Autodesk Inventor part; units mm, degrees
(part 2 of 2)
sketch "Sketch14" plane through (0, 0, 0) normal (-1, 0, 0) x (0, 0, 1)
  line L0 (-9.7925, -188.2108) -> (9.4242, -188.2108) construction
  line L1 (9.4242, -188.2108) -> (9.4242, -196.9935) construction
  line L2 (9.4242, -196.9935) -> (-9.7925, -196.9935) construction
  line L3 (-9.7925, -196.9935) -> (-9.7925, -188.2108) construction
  line L4 (-9.4479, -191.3131) -> (-8.4204, -188.2651)
  line L5 (-8.4204, -188.2651) -> (-7.9214, -188.2651)
  line L6 (-7.9214, -188.2651) -> (-6.8939, -191.3131)
  line L7 (-6.8939, -191.3131) -> (-7.3212, -191.3131)
  line L8 (-7.3212, -191.3131) -> (-7.5979, -190.461)
  line L9 (-7.5979, -190.461) -> (-8.7612, -190.461)
  line L10 (-8.7612, -190.461) -> (-9.0379, -191.3131)
  line L11 (-9.0379, -191.3131) -> (-9.4479, -191.3131)
  line L12 (-7.709, -190.1152) -> (-8.1808, -188.6801)
  line L13 (-8.1808, -188.6801) -> (-8.6501, -190.1152)
  line L14 (-8.6501, -190.1152) -> (-7.709, -190.1152)
  line L15 (-4.2461, -191.3131) -> (-4.7722, -191.3131)
  line L16 (-4.7722, -191.3131) -> (-5.7355, -190.1003)
  line L17 (-5.7355, -190.1003) -> (-6.1998, -190.1003)
  line L18 (-6.1998, -190.1003) -> (-6.1998, -191.3131)
  line L19 (-6.1998, -191.3131) -> (-6.6049, -191.3131)
  line L20 (-6.6049, -191.3131) -> (-6.6049, -188.2651)
  line L21 (-6.6049, -188.2651) -> (-5.8195, -188.2651)
  spline S0 degree 2 poles (-5.8195, -188.2651) (-5.5576, -188.2651) (-5.2044, -188.3219) (-5.0439, -188.4257) knots 0 0 0 1 2 2 2
  spline S1 degree 2 poles (-5.0439, -188.4257) (-4.8833, -188.5294) (-4.6981, -188.853) (-4.6981, -189.0926) knots 0 0 0 1 2 2 2
  spline S2 degree 2 poles (-4.6981, -189.0926) (-4.6981, -189.426) (-5.0389, -189.878) (-5.3304, -189.9867) knots 0 0 0 1 2 2 2
  line L22 (-5.3304, -189.9867) -> (-4.2461, -191.3131)
  spline S3 degree 2 poles (-5.1204, -189.1247) (-5.1204, -188.9913) (-5.2143, -188.7863) (-5.3131, -188.7196) knots 0 0 0 1 2 2 2
  spline S4 degree 2 poles (-5.3131, -188.7196) (-5.3996, -188.6628) (-5.6293, -188.6159) (-5.7972, -188.6159) knots 0 0 0 1 2 2 2
  line L23 (-5.7972, -188.6159) -> (-6.1998, -188.6159)
  line L24 (-6.1998, -188.6159) -> (-6.1998, -189.762)
  line L25 (-6.1998, -189.762) -> (-5.8442, -189.762)
  spline S5 degree 2 poles (-5.8442, -189.762) (-5.6688, -189.762) (-5.3897, -189.7002) (-5.2933, -189.6039) knots 0 0 0 1 2 2 2
  spline S6 degree 2 poles (-5.2933, -189.6039) (-5.2044, -189.5199) (-5.1204, -189.2828) (-5.1204, -189.1247) knots 0 0 0 1 2 2 2
  line L26 (-3.2926, -191.3131) -> (-3.2926, -188.6257)
  line L27 (-3.2926, -188.6257) -> (-4.3152, -188.6257)
  line L28 (-4.3152, -188.6257) -> (-4.3152, -188.2651)
  line L29 (-4.3152, -188.2651) -> (-1.865, -188.2651)
  line L30 (-1.865, -188.2651) -> (-1.865, -188.6257)
  line L31 (-1.865, -188.6257) -> (-2.8876, -188.6257)
  line L32 (-2.8876, -188.6257) -> (-2.8876, -191.3131)
  line L33 (-2.8876, -191.3131) -> (-3.2926, -191.3131)
  spline S7 degree 2 poles (-0.7065, -191.3675) (-1.0375, -191.3675) (-1.5019, -191.2291) (-1.7069, -191.1303) knots 0 0 0 1 2 2 2
  line L34 (-1.7069, -191.1303) -> (-1.7069, -190.6215)
  line L35 (-1.7069, -190.6215) -> (-1.6772, -190.6215)
  spline S8 degree 2 poles (-1.6772, -190.6215) (-1.4772, -190.8092) (-0.9708, -191.0167) (-0.7362, -191.0167) knots 0 0 0 1 2 2 2
  spline S9 degree 2 poles (-0.7362, -191.0167) (-0.4002, -191.0167) (-0.0569, -190.7376) (-0.0569, -190.5079) knots 0 0 0 1 2 2 2
  spline S10 degree 2 poles (-0.0569, -190.5079) (-0.0569, -190.3251) (-0.2372, -190.0979) (-0.4324, -190.0411) knots 0 0 0 1 2 2 2
  spline S11 degree 2 poles (-0.4324, -190.0411) (-0.5731, -190.0015) (-0.8078, -189.9472) (-0.9832, -189.9027) knots 0 0 0 1 2 2 2
  spline S12 degree 2 poles (-0.9832, -189.9027) (-1.1412, -189.8608) (-1.3907, -189.7348) (-1.4871, -189.6335) knots 0 0 0 1 2 2 2
  spline S13 degree 2 poles (-1.4871, -189.6335) (-1.5809, -189.5322) (-1.6847, -189.2605) (-1.6847, -189.0827) knots 0 0 0 1 2 2 2
  spline S14 degree 2 poles (-1.6847, -189.0827) (-1.6847, -188.7122) (-1.1067, -188.2108) (-0.6596, -188.2108) knots 0 0 0 1 2 2 2
  spline S15 degree 2 poles (-0.6596, -188.2108) (-0.4027, -188.2108) (0.0518, -188.3121) (0.2469, -188.4084) knots 0 0 0 1 2 2 2
  line L36 (0.2469, -188.4084) -> (0.2469, -188.8925)
  line L37 (0.2469, -188.8925) -> (0.2173, -188.8925)
  spline S16 degree 2 poles (0.2173, -188.8925) (0.0715, -188.7591) (-0.383, -188.5615) (-0.6324, -188.5615) knots 0 0 0 1 2 2 2
  spline S17 degree 2 poles (-0.6324, -188.5615) (-0.914, -188.5615) (-1.2623, -188.8258) (-1.2623, -189.0407) knots 0 0 0 1 2 2 2
  spline S18 degree 2 poles (-1.2623, -189.0407) (-1.2623, -189.2334) (-1.0573, -189.4631) (-0.8646, -189.515) knots 0 0 0 1 2 2 2
  spline S19 degree 2 poles (-0.8646, -189.515) (-0.7362, -189.5495) (-0.3632, -189.6385) (-0.2397, -189.6755) knots 0 0 0 1 2 2 2
  spline S20 degree 2 poles (-0.2397, -189.6755) (0.074, -189.7718) (0.3655, -190.1596) (0.3655, -190.4437) knots 0 0 0 1 2 2 2
  spline S21 degree 2 poles (0.3655, -190.4437) (0.3655, -190.624) (0.2197, -190.9698) (0.0888, -191.0908) knots 0 0 0 1 2 2 2
  spline S22 degree 2 poles (0.0888, -191.0908) (-0.0569, -191.2242) (-0.4274, -191.3675) (-0.7065, -191.3675) knots 0 0 0 1 2 2 2
  line L38 (1.808, -190.1646) -> (0.6545, -190.1646)
  line L39 (0.6545, -190.1646) -> (0.6545, -189.7941)
  line L40 (0.6545, -189.7941) -> (1.808, -189.7941)
  line L41 (1.808, -189.7941) -> (1.808, -190.1646)
  line L42 (4.0655, -191.3131) -> (2.2995, -191.3131)
  line L43 (2.2995, -191.3131) -> (2.2995, -188.2651)
  line L44 (2.2995, -188.2651) -> (2.7046, -188.2651)
  line L45 (2.7046, -188.2651) -> (2.7046, -190.9525)
  line L46 (2.7046, -190.9525) -> (4.0655, -190.9525)
  line L47 (4.0655, -190.9525) -> (4.0655, -191.3131)
  line L48 (4.0557, -191.3131) -> (5.0832, -188.2651)
  line L49 (5.0832, -188.2651) -> (5.5821, -188.2651)
  line L50 (5.5821, -188.2651) -> (6.6097, -191.3131)
  line L51 (6.6097, -191.3131) -> (6.1823, -191.3131)
  line L52 (6.1823, -191.3131) -> (5.9057, -190.461)
  line L53 (5.9057, -190.461) -> (4.7423, -190.461)
  line L54 (4.7423, -190.461) -> (4.4657, -191.3131)
  line L55 (4.4657, -191.3131) -> (4.0557, -191.3131)
  line L56 (5.7946, -190.1152) -> (5.3228, -188.6801)
  line L57 (5.3228, -188.6801) -> (4.8535, -190.1152)
  line L58 (4.8535, -190.1152) -> (5.7946, -190.1152)
  spline S23 degree 2 poles (8.9661, -190.377) (8.9661, -190.6042) (8.7932, -190.9525) (8.6499, -191.0661) knots 0 0 0 1 2 2 2
  spline S24 degree 2 poles (8.6499, -191.0661) (8.477, -191.1995) (8.0843, -191.3131) (7.773, -191.3131) knots 0 0 0 1 2 2 2
  line L59 (7.773, -191.3131) -> (6.8987, -191.3131)
  line L60 (6.8987, -191.3131) -> (6.8987, -188.2651)
  line L61 (6.8987, -188.2651) -> (7.7063, -188.2651)
  spline S25 degree 2 poles (7.7063, -188.2651) (8.0324, -188.2651) (8.3584, -188.3071) (8.5066, -188.3886) knots 0 0 0 1 2 2 2
  spline S26 degree 2 poles (8.5066, -188.3886) (8.6721, -188.4751) (8.8228, -188.7591) (8.8228, -188.9518) knots 0 0 0 1 2 2 2
  spline S27 degree 2 poles (8.8228, -188.9518) (8.8228, -189.1667) (8.5956, -189.5075) (8.3955, -189.6039) knots 0 0 0 1 2 2 2
  line L62 (8.3955, -189.6039) -> (8.3955, -189.6187)
  spline S28 degree 2 poles (8.3955, -189.6187) (8.6672, -189.6928) (8.9661, -190.0855) (8.9661, -190.377) knots 0 0 0 1 2 2 2
  spline S29 degree 2 poles (8.5437, -190.3943) (8.5437, -190.2214) (8.4449, -189.9991) (8.2967, -189.92) knots 0 0 0 1 2 2 2
  spline S30 degree 2 poles (8.2967, -189.92) (8.2004, -189.8706) (7.9731, -189.841) (7.7632, -189.841) knots 0 0 0 1 2 2 2
  line L63 (7.7632, -189.841) -> (7.3037, -189.841)
  line L64 (7.3037, -189.841) -> (7.3037, -190.9673)
  line L65 (7.3037, -190.9673) -> (7.6322, -190.9673)
  spline S31 degree 2 poles (7.6322, -190.9673) (7.899, -190.9673) (8.2053, -190.9179) (8.3239, -190.8389) knots 0 0 0 1 2 2 2
  spline S32 degree 2 poles (8.3239, -190.8389) (8.4375, -190.7574) (8.5437, -190.5548) (8.5437, -190.3943) knots 0 0 0 1 2 2 2
  spline S33 degree 2 poles (8.4004, -189.0086) (8.4004, -188.8999) (8.3263, -188.7369) (8.2448, -188.69) knots 0 0 0 1 2 2 2
  spline S34 degree 2 poles (8.2448, -188.69) (8.146, -188.6356) (7.9064, -188.6109) (7.6915, -188.6109) knots 0 0 0 1 2 2 2
  line L66 (7.6915, -188.6109) -> (7.3037, -188.6109)
  line L67 (7.3037, -188.6109) -> (7.3037, -189.5026)
  line L68 (7.3037, -189.5026) -> (7.7632, -189.5026)
  spline S35 degree 2 poles (7.7632, -189.5026) (7.9534, -189.5026) (8.1337, -189.4631) (8.23, -189.4013) knots 0 0 0 1 2 2 2
  spline S36 degree 2 poles (8.23, -189.4013) (8.3239, -189.342) (8.4004, -189.1519) (8.4004, -189.0086) knots 0 0 0 1 2 2 2
  spline S37 degree 2 poles (-7.7226, -195.3633) (-7.7226, -195.5832) (-7.8634, -195.9586) (-7.9918, -196.0969) knots 0 0 0 1 2 2 2
  spline S38 degree 2 poles (-7.9918, -196.0969) (-8.1203, -196.2352) (-8.5031, -196.3958) (-8.7403, -196.3958) knots 0 0 0 1 2 2 2
  spline S39 degree 2 poles (-8.7403, -196.3958) (-8.9576, -196.3958) (-9.3825, -196.2995) (-9.5381, -196.2229) knots 0 0 0 1 2 2 2
  line L69 (-9.5381, -196.2229) -> (-9.5381, -195.7906)
  line L70 (-9.5381, -195.7906) -> (-9.5084, -195.7906)
  spline S40 degree 2 poles (-9.5084, -195.7906) (-9.4615, -195.8252) (-9.2861, -195.9141) (-9.1799, -195.9537) knots 0 0 0 1 2 2 2
  spline S41 degree 2 poles (-9.1799, -195.9537) (-9.0589, -195.9957) (-8.8588, -196.0426) (-8.7328, -196.0426) knots 0 0 0 1 2 2 2
  spline S42 degree 2 poles (-8.7328, -196.0426) (-8.6093, -196.0426) (-8.3772, -195.9537) (-8.2932, -195.8573) knots 0 0 0 1 2 2 2
  spline S43 degree 2 poles (-8.2932, -195.8573) (-8.2166, -195.7659) (-8.1376, -195.5239) (-8.1376, -195.3609) knots 0 0 0 1 2 2 2
  spline S44 degree 2 poles (-8.1376, -195.3609) (-8.1376, -195.1978) (-8.2265, -194.9904) (-8.3105, -194.9212) knots 0 0 0 1 2 2 2
  spline S45 degree 2 poles (-8.3105, -194.9212) (-8.3969, -194.8446) (-8.6538, -194.7804) (-8.8094, -194.7804) knots 0 0 0 1 2 2 2
  spline S46 degree 2 poles (-8.8094, -194.7804) (-8.9774, -194.7804) (-9.3108, -194.8323) (-9.4121, -194.8545) knots 0 0 0 1 2 2 2
  line L71 (-9.4121, -194.8545) -> (-9.4121, -193.2836)
  line L72 (-9.4121, -193.2836) -> (-7.7399, -193.2836)
  line L73 (-7.7399, -193.2836) -> (-7.7399, -193.6417)
  line L74 (-7.7399, -193.6417) -> (-9.0194, -193.6417)
  line L75 (-9.0194, -193.6417) -> (-9.0194, -194.4544)
  spline S47 degree 2 poles (-9.0194, -194.4544) (-8.9453, -194.4445) (-8.802, -194.4371) (-8.7427, -194.4371) knots 0 0 0 1 2 2 2
  spline S48 degree 2 poles (-8.7427, -194.4371) (-8.5081, -194.4371) (-8.1845, -194.5136) (-8.0363, -194.6273) knots 0 0 0 1 2 2 2
  spline S49 degree 2 poles (-8.0363, -194.6273) (-7.8856, -194.7409) (-7.7226, -195.0867) (-7.7226, -195.3633) knots 0 0 0 1 2 2 2
  line L76 (-6.0158, -193.1477) -> (-7.2088, -196.9935)
  line L77 (-7.2088, -196.9935) -> (-7.5546, -196.9935)
  line L78 (-7.5546, -196.9935) -> (-6.3666, -193.1477)
  line L79 (-6.3666, -193.1477) -> (-6.0158, -193.1477)
  line L80 (-3.8002, -196.3316) -> (-5.6799, -196.3316)
  line L81 (-5.6799, -196.3316) -> (-5.6799, -195.8993)
  spline S50 degree 2 poles (-5.6799, -195.8993) (-5.4774, -195.7091) (-5.1167, -195.3559) (-4.9438, -195.1657) knots 0 0 0 1 2 2 2
  spline S51 degree 2 poles (-4.9438, -195.1657) (-4.5956, -194.7829) (-4.3412, -194.3235) (-4.3412, -194.0789) knots 0 0 0 1 2 2 2
  spline S52 degree 2 poles (-4.3412, -194.0789) (-4.3412, -193.9505) (-4.4202, -193.7578) (-4.4918, -193.6961) knots 0 0 0 1 2 2 2
  spline S53 degree 2 poles (-4.4918, -193.6961) (-4.5635, -193.6343) (-4.7512, -193.5726) (-4.8648, -193.5726) knots 0 0 0 1 2 2 2
  spline S54 degree 2 poles (-4.8648, -193.5726) (-4.9735, -193.5726) (-5.1958, -193.6269) (-5.2971, -193.6689) knots 0 0 0 1 2 2 2
  spline S55 degree 2 poles (-5.2971, -193.6689) (-5.3835, -193.7035) (-5.5441, -193.8023) (-5.5935, -193.8369) knots 0 0 0 1 2 2 2
  line L82 (-5.5935, -193.8369) -> (-5.6157, -193.8369)
  line L83 (-5.6157, -193.8369) -> (-5.6157, -193.4021)
  spline S56 degree 2 poles (-5.6157, -193.4021) (-5.4897, -193.3404) (-5.0377, -193.2194) (-4.8352, -193.2194) knots 0 0 0 1 2 2 2
  spline S57 degree 2 poles (-4.8352, -193.2194) (-4.4078, -193.2194) (-3.9262, -193.6714) (-3.9262, -194.0567) knots 0 0 0 1 2 2 2
  spline S58 degree 2 poles (-3.9262, -194.0567) (-3.9262, -194.237) (-4.0102, -194.5383) (-4.0843, -194.6668) knots 0 0 0 1 2 2 2
  spline S59 degree 2 poles (-4.0843, -194.6668) (-4.1584, -194.8002) (-4.3733, -195.062) (-4.4918, -195.188) knots 0 0 0 1 2 2 2
  spline S60 degree 2 poles (-4.4918, -195.188) (-4.6845, -195.3979) (-5.1563, -195.8475) (-5.2971, -195.9784) knots 0 0 0 1 2 2 2
  line L84 (-5.2971, -195.9784) -> (-3.8002, -195.9784)
  line L85 (-3.8002, -195.9784) -> (-3.8002, -196.3316)
  line L86 (-1.6661, -196.3316) -> (-3.1531, -196.3316)
  line L87 (-3.1531, -196.3316) -> (-3.1531, -196.0204)
  line L88 (-3.1531, -196.0204) -> (-2.5998, -196.0204)
  line L89 (-2.5998, -196.0204) -> (-2.5998, -193.9776)
  line L90 (-2.5998, -193.9776) -> (-3.1531, -193.9776)
  line L91 (-3.1531, -193.9776) -> (-3.1531, -193.6985)
  spline S61 degree 2 poles (-3.1531, -193.6985) (-2.8394, -193.6985) (-2.543, -193.5207) (-2.5232, -193.2737) knots 0 0 0 1 2 2 2
  line L92 (-2.5232, -193.2737) -> (-2.2071, -193.2737)
  line L93 (-2.2071, -193.2737) -> (-2.2071, -196.0204)
  line L94 (-2.2071, -196.0204) -> (-1.6661, -196.0204)
  line L95 (-1.6661, -196.0204) -> (-1.6661, -196.3316)
  line L96 (0.1617, -193.1477) -> (-1.0313, -196.9935)
  line L97 (-1.0313, -196.9935) -> (-1.3771, -196.9935)
  line L98 (-1.3771, -196.9935) -> (-0.1891, -193.1477)
  line L99 (-0.1891, -193.1477) -> (0.1617, -193.1477)
  line L100 (2.3773, -196.3316) -> (0.4976, -196.3316)
  line L101 (0.4976, -196.3316) -> (0.4976, -195.8993)
  spline S62 degree 2 poles (0.4976, -195.8993) (0.7001, -195.7091) (1.0608, -195.3559) (1.2337, -195.1657) knots 0 0 0 1 2 2 2
  spline S63 degree 2 poles (1.2337, -195.1657) (1.5819, -194.7829) (1.8364, -194.3235) (1.8364, -194.0789) knots 0 0 0 1 2 2 2
  spline S64 degree 2 poles (1.8364, -194.0789) (1.8364, -193.9505) (1.7573, -193.7578) (1.6857, -193.6961) knots 0 0 0 1 2 2 2
  spline S65 degree 2 poles (1.6857, -193.6961) (1.6141, -193.6343) (1.4263, -193.5726) (1.3127, -193.5726) knots 0 0 0 1 2 2 2
  spline S66 degree 2 poles (1.3127, -193.5726) (1.204, -193.5726) (0.9817, -193.6269) (0.8805, -193.6689) knots 0 0 0 1 2 2 2
  spline S67 degree 2 poles (0.8805, -193.6689) (0.794, -193.7035) (0.6335, -193.8023) (0.5841, -193.8369) knots 0 0 0 1 2 2 2
  line L102 (0.5841, -193.8369) -> (0.5618, -193.8369)
  line L103 (0.5618, -193.8369) -> (0.5618, -193.4021)
  spline S68 degree 2 poles (0.5618, -193.4021) (0.6878, -193.3404) (1.1398, -193.2194) (1.3424, -193.2194) knots 0 0 0 1 2 2 2
  spline S69 degree 2 poles (1.3424, -193.2194) (1.7697, -193.2194) (2.2513, -193.6714) (2.2513, -194.0567) knots 0 0 0 1 2 2 2
  spline S70 degree 2 poles (2.2513, -194.0567) (2.2513, -194.237) (2.1673, -194.5383) (2.0932, -194.6668) knots 0 0 0 1 2 2 2
  spline S71 degree 2 poles (2.0932, -194.6668) (2.0191, -194.8002) (1.8042, -195.062) (1.6857, -195.188) knots 0 0 0 1 2 2 2
  spline S72 degree 2 poles (1.6857, -195.188) (1.493, -195.3979) (1.0212, -195.8475) (0.8805, -195.9784) knots 0 0 0 1 2 2 2
  line L104 (0.8805, -195.9784) -> (2.3773, -195.9784)
  line L105 (2.3773, -195.9784) -> (2.3773, -196.3316)
  spline S73 degree 2 poles (4.6818, -194.8076) (4.6818, -195.6276) (4.2051, -196.3958) (3.7086, -196.3958) knots 0 0 0 1 2 2 2
  spline S74 degree 2 poles (3.7086, -196.3958) (3.2047, -196.3958) (2.733, -195.6128) (2.733, -194.81) knots 0 0 0 1 2 2 2
  spline S75 degree 2 poles (2.733, -194.81) (2.733, -193.9851) (3.2097, -193.2218) (3.7086, -193.2218) knots 0 0 0 1 2 2 2
  spline S76 degree 2 poles (3.7086, -193.2218) (4.21, -193.2218) (4.6818, -194.0122) (4.6818, -194.8076) knots 0 0 0 1 2 2 2
  spline S77 degree 2 poles (4.1582, -195.7363) (4.2175, -195.5856) (4.2669, -195.1213) (4.2669, -194.8076) knots 0 0 0 1 2 2 2
  spline S78 degree 2 poles (4.2669, -194.8076) (4.2669, -194.4939) (4.2175, -194.032) (4.1557, -193.8764) knots 0 0 0 1 2 2 2
  spline S79 degree 2 poles (4.1557, -193.8764) (4.094, -193.7208) (3.8791, -193.5602) (3.7086, -193.5602) knots 0 0 0 1 2 2 2
  spline S80 degree 2 poles (3.7086, -193.5602) (3.5382, -193.5602) (3.3184, -193.7208) (3.2541, -193.8813) knots 0 0 0 1 2 2 2
  spline S81 degree 2 poles (3.2541, -193.8813) (3.1924, -194.0369) (3.1479, -194.5112) (3.1479, -194.81) knots 0 0 0 1 2 2 2
  spline S82 degree 2 poles (3.1479, -194.81) (3.1479, -195.1311) (3.1875, -195.5609) (3.2517, -195.7289) knots 0 0 0 1 2 2 2
  spline S83 degree 2 poles (3.2517, -195.7289) (3.311, -195.887) (3.5308, -196.0574) (3.7086, -196.0574) knots 0 0 0 1 2 2 2
  spline S84 degree 2 poles (3.7086, -196.0574) (3.8766, -196.0574) (4.0964, -195.8969) (4.1582, -195.7363) knots 0 0 0 1 2 2 2
  line L106 (6.9518, -196.3316) -> (5.0721, -196.3316)
  line L107 (5.0721, -196.3316) -> (5.0721, -195.8993)
  spline S85 degree 2 poles (5.0721, -195.8993) (5.2746, -195.7091) (5.6352, -195.3559) (5.8081, -195.1657) knots 0 0 0 1 2 2 2
  spline S86 degree 2 poles (5.8081, -195.1657) (6.1564, -194.7829) (6.4108, -194.3235) (6.4108, -194.0789) knots 0 0 0 1 2 2 2
  spline S87 degree 2 poles (6.4108, -194.0789) (6.4108, -193.9505) (6.3318, -193.7578) (6.2602, -193.6961) knots 0 0 0 1 2 2 2
  spline S88 degree 2 poles (6.2602, -193.6961) (6.1885, -193.6343) (6.0008, -193.5726) (5.8872, -193.5726) knots 0 0 0 1 2 2 2
  spline S89 degree 2 poles (5.8872, -193.5726) (5.7785, -193.5726) (5.5562, -193.6269) (5.4549, -193.6689) knots 0 0 0 1 2 2 2
  spline S90 degree 2 poles (5.4549, -193.6689) (5.3685, -193.7035) (5.2079, -193.8023) (5.1585, -193.8369) knots 0 0 0 1 2 2 2
  line L108 (5.1585, -193.8369) -> (5.1363, -193.8369)
  line L109 (5.1363, -193.8369) -> (5.1363, -193.4021)
  spline S91 degree 2 poles (5.1363, -193.4021) (5.2623, -193.3404) (5.7143, -193.2194) (5.9168, -193.2194) knots 0 0 0 1 2 2 2
  spline S92 degree 2 poles (5.9168, -193.2194) (6.3441, -193.2194) (6.8258, -193.6714) (6.8258, -194.0567) knots 0 0 0 1 2 2 2
  spline S93 degree 2 poles (6.8258, -194.0567) (6.8258, -194.237) (6.7418, -194.5383) (6.6677, -194.6668) knots 0 0 0 1 2 2 2
  spline S94 degree 2 poles (6.6677, -194.6668) (6.5936, -194.8002) (6.3787, -195.062) (6.2602, -195.188) knots 0 0 0 1 2 2 2
  spline S95 degree 2 poles (6.2602, -195.188) (6.0675, -195.3979) (5.5957, -195.8475) (5.4549, -195.9784) knots 0 0 0 1 2 2 2
  line L110 (5.4549, -195.9784) -> (6.9518, -195.9784)
  line L111 (6.9518, -195.9784) -> (6.9518, -196.3316)
  spline S96 degree 2 poles (9.2859, -195.3436) (9.2859, -195.5782) (9.1303, -195.9759) (8.9994, -196.1093) knots 0 0 0 1 2 2 2
  spline S97 degree 2 poles (8.9994, -196.1093) (8.8636, -196.2501) (8.5227, -196.3958) (8.3177, -196.3958) knots 0 0 0 1 2 2 2
  spline S98 degree 2 poles (8.3177, -196.3958) (8.1127, -196.3958) (7.7743, -196.2575) (7.6458, -196.1192) knots 0 0 0 1 2 2 2
  spline S99 degree 2 poles (7.6458, -196.1192) (7.4878, -195.9537) (7.3099, -195.3979) (7.3099, -194.9928) knots 0 0 0 1 2 2 2
  spline S100 degree 2 poles (7.3099, -194.9928) (7.3099, -194.5952) (7.4729, -193.9554) (7.6434, -193.7183) knots 0 0 0 1 2 2 2
  spline S101 degree 2 poles (7.6434, -193.7183) (7.8089, -193.4861) (8.3325, -193.2268) (8.6758, -193.2268) knots 0 0 0 1 2 2 2
  spline S102 degree 2 poles (8.6758, -193.2268) (8.7771, -193.2268) (8.9549, -193.2465) (9.0216, -193.2688) knots 0 0 0 1 2 2 2
  line L112 (9.0216, -193.2688) -> (9.0216, -193.6615)
  line L113 (9.0216, -193.6615) -> (9.0043, -193.6615)
  spline S103 degree 2 poles (9.0043, -193.6615) (8.9475, -193.6318) (8.7401, -193.58) (8.6215, -193.58) knots 0 0 0 1 2 2 2
  spline S104 degree 2 poles (8.6215, -193.58) (8.2411, -193.58) (7.7743, -194.0937) (7.7298, -194.5976) knots 0 0 0 1 2 2 2
  spline S105 degree 2 poles (7.7298, -194.5976) (7.8755, -194.4964) (8.1818, -194.3852) (8.3646, -194.3852) knots 0 0 0 1 2 2 2
  spline S106 degree 2 poles (8.3646, -194.3852) (8.5424, -194.3852) (8.8092, -194.4568) (8.9549, -194.5655) knots 0 0 0 1 2 2 2
  spline S107 degree 2 poles (8.9549, -194.5655) (9.1229, -194.6915) (9.2859, -195.0817) (9.2859, -195.3436) knots 0 0 0 1 2 2 2
  spline S108 degree 2 poles (8.871, -195.3609) (8.871, -195.1731) (8.7722, -194.9187) (8.6635, -194.8298) knots 0 0 0 1 2 2 2
  spline S109 degree 2 poles (8.6635, -194.8298) (8.582, -194.7656) (8.3794, -194.7236) (8.2732, -194.7236) knots 0 0 0 1 2 2 2
  spline S110 degree 2 poles (8.2732, -194.7236) (8.13, -194.7236) (7.8607, -194.81) (7.7298, -194.8916) knots 0 0 0 1 2 2 2
  spline S111 degree 2 poles (7.7298, -194.8916) (7.7273, -194.936) (7.7224, -195.02) (7.7224, -195.0842) knots 0 0 0 1 2 2 2
  spline S112 degree 2 poles (7.7224, -195.0842) (7.7224, -195.4004) (7.8459, -195.7882) (7.9398, -195.8894) knots 0 0 0 1 2 2 2
  spline S113 degree 2 poles (7.9398, -195.8894) (8.0262, -195.9858) (8.2139, -196.0623) (8.3201, -196.0623) knots 0 0 0 1 2 2 2
  spline S114 degree 2 poles (8.3201, -196.0623) (8.5671, -196.0623) (8.871, -195.7116) (8.871, -195.3609) knots 0 0 0 1 2 2 2
  point P0 (0, 0)
  constraints: 2 other
emboss "Emboss2" sketch "Sketch14" operation cut depth 2.54 direction (1, 0, 0)
body "Solid1"
